Autodesk Fusion 360 part; units mm, degrees
(part 2 of 3)
sketch "Sketch3" plane through (0, -5, 0) normal (0, -1, 0) x (1, 0, 0)
  line L0 (28.5447, 14.3738) -> (28.5927, 14.6139)
  line L1 (28.5927, 14.6139) -> (28.6512, 39.9559)
  line L2 (28.6512, 39.9559) -> (28.9596, 41.1095)
  spline S0 degree 3 poles (28.9596, 41.1095) (29.1624, 41.8737) (29.4207, 42.6577) (29.7867, 43.4188) (30.0662, 43.9999) (30.3895, 44.5347) (30.7268, 45.0362) knots 0.002463 0.002463 0.002463 0.002463 0.566846 0.566846 0.566846 0.997755 0.997755 0.997755 0.997755
  spline S1 degree 3 poles (30.7268, 45.0362) (31.8623, 46.7358) (33.3627, 48.0126) (35.086, 48.9323) (35.8654, 49.3483) (36.6957, 49.6868) (37.5808, 49.9247) knots 0.001217 0.001217 0.001217 0.001217 0.688337 0.688337 0.688337 0.9991 0.9991 0.9991 0.9991
  spline S2 degree 3 poles (37.5809, 49.9247) (38.1393, 50.0755) (38.9538, 50.2376) (39.748, 50.2925) (40.2008, 50.3238) (40.6623, 50.3378) (41.2195, 50.3427) knots 0 0 0 0 0.456967 0.456967 0.456967 0.717487 0.717487 0.717487 0.717487
  line L3 (43.2375, 50.3785) -> (64.2895, 50.3304)
  spline S3 degree 3 poles (64.2895, 50.3304) (69.3375, 50.3217) (71.8718, 50.3178) (73.2853, 50.2995) (73.992, 50.2904) (74.4136, 50.2812) (74.8445, 50.2498) (75.1344, 50.2286) (75.4759, 50.185) (75.7431, 50.1318) (75.8658, 50.1074) (75.9593, 50.0853) (76.0131, 50.0726) knots 0 0 0 0 0.5 0.5 0.5 0.75 0.75 0.75 0.918213 0.918213 0.918213 0.99543 0.99543 0.99543 0.99543
  spline S4 degree 3 poles (76.0131, 50.0726) (78.7497, 49.4373) (81.2312, 47.9496) (82.9657, 45.7927) (83.8624, 44.6776) (84.5567, 43.3962) (85.0168, 42.022) (85.0171, 42.0211) (85.0175, 42.0201) (85.0178, 42.0192) knots 0.000788 0.000788 0.000788 0.000788 0.659473 0.659473 0.659473 1 1 1 1.000365 1.000365 1.000365 1.000365
  spline S5 degree 3 poles (85.0178, 42.0192) (85.0181, 42.0182) (85.0184, 42.0173) (85.0187, 42.0163) (85.0516, 41.9176) (85.1158, 41.7567) (85.2177, 41.4143) (85.3321, 41.0296) (85.439, 40.5049) (85.4918, 40.0367) (85.5914, 39.1525) (85.6029, 38.2865) (85.6162, 36.5721) (85.6311, 34.6649) (85.6279, 31.7431) (85.6279, 27.0233) knots -0.000791 -0.000791 -0.000791 -0.000791 0 0 0 0.151411 0.151411 0.151411 0.321524 0.321524 0.321524 0.642699 0.642699 0.642699 1 1 1 1
  spline S6 degree 3 poles (85.6279, 27.0233) (85.6279, 23.1991) (85.6318, 20.2771) (85.6408, 18.2245) (85.6454, 17.1759) (85.6514, 16.3534) (85.6586, 15.7622) (85.664, 15.321) (85.6707, 15.0001) (85.6757, 14.8547) (85.6761, 14.8429) (85.6765, 14.8324) (85.6768, 14.8233) knots 0 0 0 0 0.473518 0.473518 0.473518 0.715422 0.715422 0.715422 0.895914 0.895914 0.895914 0.91057 0.91057 0.91057 0.91057
  spline S7 degree 3 poles (85.6768, 14.8233) (85.78, 13.825) (86.1372, 12.4963) (86.5583, 11.5465) (86.6077, 11.435) (86.6576, 11.3286) (86.707, 11.2286) knots 0.016663 0.016663 0.016663 0.016663 0.893157 0.893157 0.893157 0.99609 0.99609 0.99609 0.99609
  spline S8 degree 3 poles (86.707, 11.2286) (87.0043, 10.6397) (87.1373, 10.444) (87.4643, 10.0658) (87.4655, 10.0645) (87.4666, 10.0631) (87.4678, 10.0618) knots 0.006764 0.006764 0.006764 0.006764 1 1 1 1.002067 1.002067 1.002067 1.002067
  spline S9 degree 3 poles (87.4678, 10.0618) (87.4689, 10.0605) (87.4701, 10.0591) (87.4712, 10.0578) (88.1686, 9.2476) (88.815, 8.3206) (89.28, 7.2967) (89.5333, 6.7388) (89.7284, 6.1697) (89.8772, 5.6188) (89.8788, 5.6129) (89.8804, 5.607) (89.882, 5.6011) knots -0.001455 -0.001455 -0.001455 -0.001455 0 0 0 0.647342 0.647342 0.647342 1 1 1 1.005845 1.005845 1.005845 1.005845
  spline S10 degree 3 poles (89.882, 5.6011) (89.8836, 5.5951) (89.8851, 5.5892) (89.8867, 5.5833) (89.9571, 5.3137) (90.0431, 4.9596) (90.1002, 4.5568) (90.1621, 4.1205) (90.1782, 3.7263) (90.185, 3.3701) (90.1876, 3.2384) (90.1889, 3.1062) (90.1899, 2.9643) (90.19, 2.959) (90.19, 2.9537) (90.19, 2.9484) knots -0.011583 -0.011583 -0.011583 -0.011583 0 0 0 0.402629 0.402629 0.402629 0.838702 0.838702 0.838702 1 1 1 1.006483 1.006483 1.006483 1.006483
  spline S11 degree 3 poles (90.19, 2.9484) (90.19, 2.9431) (90.19, 2.9377) (90.19, 2.9324) (90.19, 2.4687) (90.1909, 2.0734) (90.1389, 1.562) (90.0975, 1.1547) (90.0104, 0.7153) (89.9283, 0.3949) knots -0.006925 -0.006925 -0.006925 -0.006925 0 0 0 0.554445 0.554445 0.554445 0.995951 0.995951 0.995951 0.995951
  spline S12 degree 3 poles (89.9283, 0.3949) (89.2588, -2.2434) (87.6414, -4.4379) (85.5824, -5.8498) (83.3601, -7.3736) (80.5963, -8.0488) (77.8293, -7.5933) (76.6106, -7.3927) (75.3981, -6.9683) (74.2734, -6.3206) (74.2714, -6.3195) (74.2694, -6.3184) (74.2674, -6.3172) knots 0.000423 0.000423 0.000423 0.000423 0.3917 0.3917 0.3917 0.814004 0.814004 0.814004 1 1 1 1.000565 1.000565 1.000565 1.000565
  spline S13 degree 3 poles (74.2674, -6.3172) (74.2655, -6.316) (74.2635, -6.3149) (74.2615, -6.3137) (73.6843, -5.979) (72.7241, -5.6295) (71.6961, -5.4737) (71.6954, -5.4736) (71.6947, -5.4735) (71.694, -5.4734) knots -0.00171 -0.00171 -0.00171 -0.00171 0 0 0 1 1 1 1.000449 1.000449 1.000449 1.000449
  spline S14 degree 3 poles (71.694, -5.4734) (71.6933, -5.4733) (71.6927, -5.4732) (71.692, -5.4731) (71.4636, -5.4383) (71.3375, -5.4212) (70.8719, -5.3978) (69.9429, -5.351) (67.867, -5.3283) (63.1123, -5.3297) (61.2764, -5.3303) (59.0354, -5.3336) (56.2884, -5.3383) (56.2882, -5.3383) (56.2879, -5.3383) (56.2877, -5.3383) knots -0.000531 -0.000531 -0.000531 -0.000531 0 0 0 0.265563 0.265563 0.265563 0.795413 0.795413 0.795413 1 1 1 1.000016 1.000016 1.000016 1.000016
  spline S15 degree 3 poles (56.2877, -5.3383) (56.2875, -5.3383) (56.2873, -5.3383) (56.2871, -5.3383) (49.133, -5.3487) (45.769, -5.3576) (44.1594, -5.38) (43.3075, -5.3919) (42.958, -5.4118) (42.9119, -5.4159) (42.911, -5.416) (42.9103, -5.416) (42.9096, -5.4161) knots -0.000018 -0.000018 -0.000018 -0.000018 0 0 0 0.595196 0.595196 0.595196 0.910216 0.910216 0.910216 0.916088 0.916088 0.916088 0.916088
  spline S16 degree 3 poles (42.9096, -5.4161) (41.5575, -5.6043) (40.5785, -5.9576) (39.93, -6.3379) (39.9283, -6.3389) (39.9266, -6.3399) (39.9249, -6.3409) knots 0.005759 0.005759 0.005759 0.005759 1 1 1 1.001321 1.001321 1.001321 1.001321
  spline S17 degree 3 poles (39.9249, -6.3409) (39.9232, -6.3419) (39.9215, -6.3428) (39.9198, -6.3438) (38.3615, -7.2521) (36.7048, -7.6682) (34.9959, -7.7237) (34.5397, -7.7385) (34.079, -7.7249) (33.6144, -7.6795) knots -0.001663 -0.001663 -0.001663 -0.001663 0 0 0 0.789303 0.789303 0.789303 1 1 1 1
  spline S18 degree 3 poles (33.6144, -7.6795) (31.0087, -7.4269) (28.7159, -6.2217) (27.0024, -4.4425) (25.9971, -3.3987) (25.1834, -2.1388) (24.6669, -0.7013) (24.6659, -0.6984) (24.6649, -0.6956) (24.6639, -0.6927) knots 0.000439 0.000439 0.000439 0.000439 0.630416 0.630416 0.630416 1 1 1 1.001322 1.001322 1.001322 1.001322
  spline S19 degree 3 poles (24.6639, -0.6927) (23.792, 1.7499) (23.8315, 4.463) (24.7752, 6.841) (25.2611, 8.0655) (25.9744, 9.1996) (26.8664, 10.1907) (26.8665, 10.1908) (26.8666, 10.1909) (26.8668, 10.1911) knots 0 0 0 0 0.660104 0.660104 0.660104 1 1 1 1.000071 1.000071 1.000071 1.000071
  spline S20 degree 3 poles (26.8668, 10.1911) (26.8669, 10.1912) (26.867, 10.1913) (26.8671, 10.1914) (27.2467, 10.6131) (27.8393, 11.6247) (28.2707, 13.2034) (28.3696, 13.5653) (28.4615, 13.9552) (28.5441, 14.3711) (28.5443, 14.372) (28.5445, 14.3729) (28.5447, 14.3738) knots -0.000091 -0.000091 -0.000091 -0.000091 0 0 0 0.813499 0.813499 0.813499 1 1 1 1.000326 1.000326 1.000326 1.000326
  line L4 (28.1853, 41.3106) -> (27.8515, 40.0619)
  line L5 (27.8515, 40.0619) -> (27.7929, 14.694)
  line L6 (27.7929, 14.694) -> (27.7601, 14.5302)
  spline S21 degree 3 poles (27.7601, 14.5302) (27.7599, 14.5292) (27.7597, 14.5281) (27.7595, 14.5271) (27.6479, 13.9658) (27.5196, 13.4579) (27.3817, 13.0097) (26.9944, 11.7509) (26.5124, 10.993) (26.2726, 10.7267) (26.2725, 10.7266) (26.2723, 10.7264) (26.2722, 10.7263) knots -1.000384 -1.000384 -1.000384 -1.000384 -1 -1 -1 -0.737392 -0.737392 -0.737392 0 0 0 0.000107 0.000107 0.000107 0.000107
  spline S22 degree 3 poles (26.2722, 10.7263) (26.272, 10.7261) (26.2719, 10.726) (26.2718, 10.7258) (25.2452, 9.5852) (24.4359, 8.2609) (23.9141, 6.8271) (23.0115, 4.3472) (23.0138, 1.5501) (23.9104, -0.9616) (23.911, -0.9633) (23.9116, -0.965) (23.9122, -0.9667) knots -1.000083 -1.000083 -1.000083 -1.000083 -1 -1 -1 -0.633646 -0.633646 -0.633646 0 0 0 0.000763 0.000763 0.000763 0.000763
  spline S23 degree 3 poles (23.9122, -0.9667) (23.9128, -0.9684) (23.9134, -0.9701) (23.9141, -0.9718) (24.5193, -2.6566) (25.4993, -4.1093) (26.7116, -5.2837) (28.5164, -7.0321) (30.8677, -8.2168) (33.5366, -8.4758) knots -1.000779 -1.000779 -1.000779 -1.000779 -1 -1 -1 -0.598384 -0.598384 -0.598384 -0.000479 -0.000479 -0.000479 -0.000479
  spline S24 degree 3 poles (33.5366, -8.4758) (34.1121, -8.532) (34.6806, -8.5429) (35.2421, -8.5141) (36.9979, -8.4238) (38.6981, -7.9819) (40.3227, -7.035) (40.3247, -7.0338) (40.3267, -7.0327) (40.3287, -7.0315) knots -1 -1 -1 -1 -0.757667 -0.757667 -0.757667 0 0 0 0.001959 0.001959 0.001959 0.001959
  spline S25 degree 3 poles (40.3287, -7.0315) (40.3307, -7.0303) (40.3327, -7.0292) (40.3346, -7.028) (40.8689, -6.7147) (41.7382, -6.3892) (42.9969, -6.2117) knots -1.001555 -1.001555 -1.001555 -1.001555 -1 -1 -1 -0.011769 -0.011769 -0.011769 -0.011769
  spline S26 degree 3 poles (42.9969, -6.2117) (43.0795, -6.2058) (43.4713, -6.1887) (44.3196, -6.178) (45.9764, -6.157) (49.3494, -6.1484) (56.2883, -6.1383) (56.2885, -6.1383) (56.2888, -6.1383) (56.289, -6.1383) knots -0.872881 -0.872881 -0.872881 -0.872881 -0.57731 -0.57731 -0.57731 0 0 0 0.000021 0.000021 0.000021 0.000021
  spline S27 degree 3 poles (56.289, -6.1383) (56.2893, -6.1383) (56.2895, -6.1383) (56.2898, -6.1383) (59.3936, -6.1329) (61.8513, -6.1294) (63.8076, -6.1296) (68.0415, -6.1301) (69.9643, -6.1538) (70.8167, -6.196) (71.2742, -6.2187) (71.3614, -6.232) (71.5714, -6.264) (71.5722, -6.2641) (71.573, -6.2642) (71.5738, -6.2644) knots -1.000018 -1.000018 -1.000018 -1.000018 -1 -1 -1 -0.768828 -0.768828 -0.768828 -0.268512 -0.268512 -0.268512 0 0 0 0.000626 0.000626 0.000626 0.000626
  spline S28 degree 3 poles (71.5738, -6.2644) (71.5746, -6.2645) (71.5754, -6.2646) (71.5763, -6.2647) (72.5139, -6.4068) (73.3872, -6.7315) (73.8601, -7.0058) (73.8624, -7.0071) (73.8648, -7.0085) (73.8671, -7.0098) knots -1.000529 -1.000529 -1.000529 -1.000529 -1 -1 -1 0 0 0 0.002014 0.002014 0.002014 0.002014
  spline S29 degree 3 poles (73.8671, -7.0098) (73.8695, -7.0112) (73.8718, -7.0125) (73.8742, -7.0139) (75.2779, -7.8223) (76.8124, -8.3068) (78.3374, -8.4691) (81.2395, -8.778) (84.0823, -7.9571) (86.3566, -6.2808) (88.4137, -4.7645) (90.0207, -2.4927) (90.7035, 0.1972) knots -1.000666 -1.000666 -1.000666 -1.000666 -1 -1 -1 -0.783863 -0.783863 -0.783863 -0.372519 -0.372519 -0.372519 -0.000464 -0.000464 -0.000464 -0.000464
  spline S30 degree 3 poles (90.7035, 0.1972) (90.7945, 0.5524) (90.894, 1.0612) (90.9385, 1.5182) (90.9918, 2.0648) (90.99, 2.4724) (90.99, 2.9324) (90.99, 2.9387) (90.99, 2.945) (90.99, 2.9512) knots -0.995571 -0.995571 -0.995571 -0.995571 -0.542171 -0.542171 -0.542171 0 0 0 0.008156 0.008156 0.008156 0.008156
  spline S31 degree 3 poles (90.99, 2.9512) (90.99, 2.9575) (90.9899, 2.9637) (90.9899, 2.97) (90.9887, 3.1396) (90.9871, 3.2972) (90.9833, 3.46) (90.9752, 3.8126) (90.9554, 4.2319) (90.8895, 4.6883) (90.8262, 5.1272) (90.733, 5.5087) (90.6607, 5.7856) (90.6588, 5.7926) (90.657, 5.7996) (90.6552, 5.8065) knots -1.007635 -1.007635 -1.007635 -1.007635 -1 -1 -1 -0.809537 -0.809537 -0.809537 -0.396848 -0.396848 -0.396848 0 0 0 0.013642 0.013642 0.013642 0.013642
  spline S32 degree 3 poles (90.6552, 5.8065) (90.6533, 5.8135) (90.6514, 5.8205) (90.6495, 5.8275) (90.4769, 6.4667) (90.2416, 7.1395) (89.9313, 7.7935) (89.436, 8.8374) (88.7711, 9.7739) (88.0776, 10.5797) (88.0762, 10.5813) (88.0749, 10.5828) (88.0735, 10.5844) knots -1.006884 -1.006884 -1.006884 -1.006884 -1 -1 -1 -0.61483 -0.61483 -0.61483 0 0 0 0.001713 0.001713 0.001713 0.001713
  spline S33 degree 3 poles (88.0735, 10.5844) (88.0721, 10.586) (88.0708, 10.5876) (88.0694, 10.5891) (88.0403, 10.6228) (88.0135, 10.6546) (87.9887, 10.6847) (87.7701, 10.9505) (87.6698, 11.0971) (87.4227, 11.5861) knots -1.002435 -1.002435 -1.002435 -1.002435 -1 -1 -1 -0.898949 -0.898949 -0.898949 -0.008653 -0.008653 -0.008653 -0.008653
  spline S34 degree 3 poles (87.4227, 11.5861) (87.3635, 11.706) (87.3027, 11.838) (87.2426, 11.9789) (86.8785, 12.8313) (86.5675, 14.0165) (86.4753, 14.8796) knots -0.994911 -0.994911 -0.994911 -0.994911 -0.857358 -0.857358 -0.857358 -0.025015 -0.025015 -0.025015 -0.025015
  spline S35 degree 3 poles (86.4753, 14.8796) (86.4752, 14.8824) (86.4751, 14.8853) (86.475, 14.8883) (86.4703, 15.028) (86.4636, 15.3508) (86.4583, 15.7942) (86.4511, 16.388) (86.4452, 17.2152) (86.4406, 18.269) (86.4318, 20.3172) (86.4279, 23.225) (86.4279, 27.0233) knots -0.896967 -0.896967 -0.896967 -0.896967 -0.893105 -0.893105 -0.893105 -0.712378 -0.712378 -0.712378 -0.470371 -0.470371 -0.470371 0 0 0 0
  spline S36 degree 3 poles (86.4279, 27.0233) (86.4279, 32.0037) (86.4315, 34.9791) (86.4136, 36.8869) (86.3986, 38.4761) (86.3894, 39.3) (86.2734, 40.2394) (86.2125, 40.7327) (86.0879, 41.3033) (85.9679, 41.6972) (85.8632, 42.0409) (85.8042, 42.1896) (85.7777, 42.2693) (85.7773, 42.2704) (85.7769, 42.2715) (85.7766, 42.2727) knots -1 -1 -1 -1 -0.622947 -0.622947 -0.622947 -0.308857 -0.308857 -0.308857 -0.143922 -0.143922 -0.143922 0 0 0 0.000931 0.000931 0.000931 0.000931
  spline S37 degree 3 poles (85.7766, 42.2727) (85.7762, 42.2738) (85.7758, 42.2749) (85.7754, 42.276) (85.2484, 43.8501) (84.4288, 45.3154) (83.3624, 46.568) (81.5254, 48.7257) (78.9721, 50.2067) (76.1953, 50.8516) knots -1.00043 -1.00043 -1.00043 -1.00043 -1 -1 -1 -0.63304 -0.63304 -0.63304 -0.000881 -0.000881 -0.000881 -0.000881
  spline S38 degree 3 poles (76.1953, 50.8516) (76.1292, 50.8672) (75.9985, 50.898) (75.8301, 50.9298) (75.5363, 50.9854) (75.1922, 51.0265) (74.9027, 51.0476) (74.4377, 51.0816) (74.008, 51.0902) (73.2956, 51.0994) (71.8708, 51.1179) (69.3389, 51.1217) (64.2909, 51.1304) knots -0.994872 -0.994872 -0.994872 -0.994872 -0.905652 -0.905652 -0.905652 -0.75 -0.75 -0.75 -0.5 -0.5 -0.5 0 0 0 0
  line L7 (64.2909, 51.1304) -> (41.3067, 51.183)
  spline S39 degree 3 poles (40.09, 51.1135) (39.9226, 51.1058) (39.7579, 51.0959) (39.592, 51.0832) (38.7865, 51.022) (37.9297, 50.8475) (37.3724, 50.6971) knots -0.529015 -0.529015 -0.529015 -0.529015 -0.438651 -0.438651 -0.438651 0 0 0 0
  spline S40 degree 3 poles (37.3724, 50.6971) (36.3395, 50.4194) (35.3819, 50.0162) (34.4897, 49.5182) (32.7505, 48.5474) (31.2338, 47.2348) (30.0622, 45.4817) knots -0.999011 -0.999011 -0.999011 -0.999011 -0.660747 -0.660747 -0.660747 -0.001343 -0.001343 -0.001343 -0.001343
  spline S41 degree 3 poles (30.0622, 45.4817) (29.7101, 44.9579) (29.3636, 44.3856) (29.0632, 43.7602) (28.6708, 42.9432) (28.3952, 42.1024) (28.1853, 41.3106) knots -0.997484 -0.997484 -0.997484 -0.997484 -0.565614 -0.565614 -0.565614 -0.001492 -0.001492 -0.001492 -0.001492
  line L8 (42.0053, 0) -> (48.0053, 0)
  line L9 (48.0053, 0) -> (48.0053, -5.8307)
  line L10 (48.0053, -5.8307) -> (42.0053, -5.8307)
  line L11 (42.0053, -5.8307) -> (42.0053, 0)
  line L12 (72, 0) -> (66, 0)
  line L13 (66, 0) -> (66, -6)
  line L14 (66, -6) -> (72, -6)
  line L15 (72, -6) -> (72, 0)
  line L16 (80.6865, 13.92) -> (86.435, 13.92)
  line L17 (86.435, 13.92) -> (86.435, 19.92)
  line L18 (86.435, 19.92) -> (80.6865, 19.92)
  line L19 (80.6865, 19.92) -> (80.6865, 13.92)
  line L20 (80.6865, 38.9642) -> (86.1487, 38.9642)
  line L21 (86.1487, 38.9642) -> (86.1487, 32.9642)
  line L22 (86.1487, 32.9642) -> (80.6865, 32.9642)
  line L23 (80.6865, 32.9642) -> (80.6865, 38.9642)
  line L24 (74.3465, 45.2067) -> (68.3465, 45.2067)
  line L25 (68.3465, 45.2067) -> (68.3465, 50.5)
  line L26 (68.3465, 50.5) -> (74.3465, 50.5)
  line L27 (74.3465, 50.5) -> (74.3465, 45.2067)
  line L28 (54.0984, 45.8537) -> (60.0984, 45.8537)
  line L29 (60.0984, 45.8537) -> (60.0984, 50.5)
  line L30 (60.0984, 50.5) -> (54.0984, 50.5)
  line L31 (54.0984, 50.5) -> (54.0984, 45.8537)
  line L32 (45, 45.5) -> (39, 45.5)
  line L33 (39, 45.5) -> (39, 50.5)
  line L34 (39, 50.5) -> (45, 50.5)
  line L35 (45, 50.5) -> (45, 45.5)
  line L36 (34, 14.228) -> (28.2082, 14.228)
  line L37 (28.2082, 14.228) -> (28.2082, 20.228)
  line L38 (28.2082, 20.228) -> (34, 20.228)
  line L39 (34, 20.228) -> (34, 14.228)
  line L40 (33.5917, 38.2953) -> (28.2286, 38.2953)
  line L41 (28.2286, 38.2953) -> (28.2286, 32.2953)
  line L42 (28.2286, 32.2953) -> (33.5917, 32.2953)
  line L43 (33.5917, 32.2953) -> (33.5917, 38.2953)
  line L44 (41.2195, 50.3427) -> (43.2375, 50.3785)
  line L45 (41.3067, 51.183) -> (40.09, 51.1135)
  point P0 (54.0984, 45.8537)
  dimension "d7" = 6
  dimension "d8" = 6
  dimension "d9" = 6
  dimension "d10" = 6
  dimension "d11" = 6
  dimension "d12" = 6
  dimension "d13" = 6
  dimension "d14" = 6
  dimension "d15" = 6
  constraint horizontal L8
  constraint vertical L9
  constraint horizontal L10
  constraint vertical L11
  constraint horizontal L12
  constraint vertical L13
  constraint horizontal L14
  constraint vertical L15
  constraint horizontal L16
  constraint vertical L17
  constraint horizontal L18
  constraint vertical L19
  constraint coincident S35 L17.end
  constraint horizontal L20
  constraint vertical L21
  constraint horizontal L22
  constraint vertical L23
  constraint horizontal L24
  constraint vertical L25
  constraint horizontal L26
  constraint vertical L27
  constraint horizontal L28
  constraint vertical L29
  constraint horizontal L30
  constraint vertical L31
  constraint coincident P0 L28.start
  constraint horizontal L32
  constraint vertical L33
  constraint horizontal L34
  constraint vertical L35
  constraint horizontal L36
  constraint vertical L37
  constraint horizontal L38
  constraint vertical L39
  constraint horizontal L40
  constraint vertical L41
  constraint horizontal L42
  constraint vertical L43
  measures "d7" distance of L12.start L12.end
  measures "d8" distance of L8.start L8.end
  measures "d9" distance of L20.start L22.end
  measures "d10" distance of L16.end L17.end
  measures "d11" distance of L24.start L24.end
  measures "d12" distance of P0 L28.end
  measures "d13" distance of L32.start L32.end
  measures "d14" distance of L40.start L42.end
  measures "d15" distance of L36.start L38.end
extrude "Extrude3" add sketch "Sketch3" 1 faces at (81.3493, -5, 2.502) along normal blind 7 contours L0 L1 S20 L36 L37 L38 | L0 L1 S20 L36 L38 L39 | L4 L5 L6 S21 S22 S23 S24 S25 S26 S27 S28 S29 S30 S31 S32 S33 S34 S35 S36 S37 S38 L7 S39 S40 S41 L45 | L1 L40 L41 L42 | L1 L40 L42 L43 | S15 S16 L8 L9 L11 | S15 S16 L9 L10 L11 | S2 L3 L33 L34 L35 L44 | S2 L3 L32 L33 L35 L44 | S13 S14 L12 L13 L15 | S13 S14 L13 L14 L15 | L3 L29 L30 L31 | L3 L28 L29 L31 | S3 L25 L26 L27 | S3 L24 L25 L27 | S6 S7 L16 L18 L19 | S6 S7 L16 L17 L18 | S5 L20 L21 L22 | S5 L20 L22 L23 on bodies 3 bodies 2 3
sketch "Sketch6" plane through (0, -12, 0) normal (0, -1, 0) x (1, 0, 0)
  line L0 (33.1474, 38.2953) -> (28.6474, 38.2953)
  line L1 (28.6474, 38.2953) -> (28.6512, 39.9559)
  line L2 (28.6512, 39.9559) -> (28.9596, 41.1095)
  spline S0 degree 3 poles (28.9596, 41.1095) (29.1624, 41.8737) (29.4207, 42.6577) (29.7867, 43.4188) (30.0662, 43.9999) (30.3895, 44.5347) (30.7268, 45.0362) knots 0.002463 0.002463 0.002463 0.002463 0.566846 0.566846 0.566846 0.997755 0.997755 0.997755 0.997755
  spline S1 degree 3 poles (30.7268, 45.0362) (31.8623, 46.7358) (33.3627, 48.0126) (35.086, 48.9323) (35.8654, 49.3483) (36.6957, 49.6868) (37.5808, 49.9247) knots 0.001217 0.001217 0.001217 0.001217 0.688337 0.688337 0.688337 0.9991 0.9991 0.9991 0.9991
  spline S2 degree 3 poles (37.5809, 49.9247) (37.9634, 50.028) (38.466, 50.1366) (39, 50.2124) knots 0 0 0 0 0.313008 0.313008 0.313008 0.313008
  line L3 (39, 50.2124) -> (39, 45.6439)
  spline S3 degree 3 poles (39, 45.6439) (38.9203, 45.6244) (38.839, 45.6033) (38.7536, 45.5802) knots -0.090057 -0.090057 -0.090057 -0.090057 0 0 0 0
  spline S4 degree 3 poles (38.7536, 45.5802) (37.0603, 45.1263) (35.4193, 43.9625) (34.465, 42.531) knots -1 -1 -1 -1 0 0 0 0
  spline S5 degree 3 poles (34.465, 42.531) (33.8656, 41.6407) (33.5921, 41.0239) (33.307, 39.9474) knots -1 -1 -1 -1 0 0 0 0
  line L4 (33.307, 39.9474) -> (33.1499, 39.3597)
  line L5 (33.1499, 39.3597) -> (33.1474, 38.2953)
  line L6 (33.1335, 32.2953) -> (33.1057, 20.228)
  line L7 (33.1057, 20.228) -> (28.6057, 20.228)
  line L8 (28.6057, 20.228) -> (28.6335, 32.2953)
  line L9 (28.6335, 32.2953) -> (33.1335, 32.2953)
  line L10 (45, 45.8223) -> (45, 50.3745)
  line L11 (45, 50.3745) -> (54.0984, 50.3537)
  line L12 (54.0984, 50.3537) -> (54.0984, 45.8537)
  line L13 (54.0984, 45.8537) -> (60.0984, 45.8537)
  line L14 (60.0984, 45.8537) -> (60.0984, 50.34)
  line L15 (60.0984, 50.34) -> (64.2895, 50.3304)
  spline S6 degree 3 poles (64.2895, 50.3304) (65.8756, 50.3277) (67.2135, 50.3254) (68.3465, 50.323) knots 0 0 0 0 0.157099 0.157099 0.157099 0.157099
  line L16 (68.3465, 50.323) -> (68.3465, 45.8229)
  spline S7 degree 3 poles (68.3465, 45.8229) (67.2123, 45.8254) (65.8709, 45.8277) (64.2818, 45.8304) knots -0.157407 -0.157407 -0.157407 -0.157407 0 0 0 0
  line L17 (64.2818, 45.8304) -> (54.0984, 45.8537)
  line L18 (54.0984, 45.8537) -> (55.6987, 44.2477)
  line L19 (55.6987, 44.2477) -> (57.2989, 42.6474)
  line L20 (57.2989, 42.6474) -> (63.3391, 42.6474)
  line L21 (63.3391, 42.6474) -> (60.2608, 39.5517)
  spline S8 degree 3 poles (60.2608, 39.5517) (58.5733, 37.8467) (57.1651, 36.4385) (57.136, 36.4269) knots -1 -1 -1 -1 0 0 0 0
  spline S9 degree 3 poles (57.136, 36.4269) (57.1069, 36.4152) (55.1808, 38.3064) (52.8531, 40.6224) knots -1 -1 -1 -1 0 0 0 0
  spline S10 degree 3 poles (52.8531, 40.6224) (50.5313, 42.9442) (48.5063, 44.9285) (48.3492, 45.0274) knots -1 -1 -1 -1 0 0 0 0
  spline S11 degree 3 poles (48.3492, 45.0274) (47.9884, 45.2718) (47.4298, 45.5278) (46.9352, 45.685) knots -1 -1 -1 -1 0 0 0 0
  spline S12 degree 3 poles (46.9352, 45.685) (46.6336, 45.7809) (46.4863, 45.8051) (45, 45.8223) knots -1 -1 -1 -1 -0.214752 -0.214752 -0.214752 -0.214752
  line L22 (74.3465, 45.772) -> (74.3465, 50.277)
  spline S13 degree 3 poles (74.3465, 50.277) (74.5216, 50.2703) (74.6824, 50.2616) (74.8445, 50.2498) (75.1344, 50.2286) (75.4759, 50.185) (75.7431, 50.1318) (75.8658, 50.1074) (75.9593, 50.0853) (76.0131, 50.0726) knots 0.655951 0.655951 0.655951 0.655951 0.75 0.75 0.75 0.918213 0.918213 0.918213 0.99543 0.99543 0.99543 0.99543
  spline S14 degree 3 poles (76.0131, 50.0726) (78.7497, 49.4373) (81.2312, 47.9496) (82.9657, 45.7927) (83.8624, 44.6776) (84.5567, 43.3962) (85.0168, 42.022) (85.0171, 42.0211) (85.0175, 42.0201) (85.0178, 42.0192) knots 0.000788 0.000788 0.000788 0.000788 0.659473 0.659473 0.659473 1 1 1 1.000365 1.000365 1.000365 1.000365
  spline S15 degree 3 poles (85.0178, 42.0192) (85.0181, 42.0182) (85.0184, 42.0173) (85.0187, 42.0163) (85.0516, 41.9176) (85.1158, 41.7567) (85.2177, 41.4143) (85.3321, 41.0296) (85.439, 40.5049) (85.4918, 40.0367) (85.5305, 39.6934) (85.5559, 39.3528) (85.5733, 38.9642) knots -0.000791 -0.000791 -0.000791 -0.000791 0 0 0 0.151411 0.151411 0.151411 0.321524 0.321524 0.321524 0.446232 0.446232 0.446232 0.446232
  line L23 (85.5733, 38.9642) -> (81.0642, 38.9642)
  spline S16 degree 3 poles (81.0642, 38.9642) (81.0123, 39.9434) (80.9185, 40.0867) (80.7497, 40.5933) knots -0.420598 -0.420598 -0.420598 -0.420598 0 0 0 0
  spline S17 degree 3 poles (80.7497, 40.5933) (79.8768, 43.2002) (77.8052, 45.039) (74.9888, 45.6908) knots -1 -1 -1 -1 0 0 0 0
  spline S18 degree 3 poles (74.9888, 45.6908) (74.8321, 45.7278) (74.7143, 45.7535) (74.3465, 45.772) knots -1 -1 -1 -1 -0.697416 -0.697416 -0.697416 -0.697416
  line L24 (81.1275, 32.9642) -> (85.6275, 32.9642)
  spline S19 degree 3 poles (85.6275, 32.9642) (85.6287, 31.3852) (85.6279, 29.4399) (85.6279, 27.0233) knots 0.817055 0.817055 0.817055 0.817055 1 1 1 1
  spline S20 degree 3 poles (85.6279, 27.0233) (85.6279, 24.1513) (85.6301, 21.7882) (85.635, 19.92) knots 0 0 0 0 0.355613 0.355613 0.355613 0.355613
  line L25 (85.635, 19.92) -> (81.135, 19.92)
  spline S21 degree 3 poles (81.135, 19.92) (81.1301, 21.793) (81.1279, 24.1549) (81.1279, 27.0233) knots -0.354876 -0.354876 -0.354876 -0.354876 0 0 0 0
  spline S22 degree 3 poles (81.1279, 27.0233) (81.1279, 29.4417) (81.1287, 31.3891) (81.1275, 32.9642) knots -1 -1 -1 -1 -0.816995 -0.816995 -0.816995 -0.816995
  line L26 (81.2537, 13.92) -> (85.8196, 13.92)
  spline S23 degree 3 poles (85.8196, 13.92) (85.9856, 13.1087) (86.2554, 12.2296) (86.5583, 11.5465) (86.6077, 11.435) (86.6576, 11.3286) (86.707, 11.2286) knots 0.262747 0.262747 0.262747 0.262747 0.893157 0.893157 0.893157 0.99609 0.99609 0.99609 0.99609
  spline S24 degree 3 poles (86.707, 11.2286) (87.0043, 10.6397) (87.1373, 10.444) (87.4643, 10.0658) (87.4655, 10.0645) (87.4666, 10.0631) (87.4678, 10.0618) knots 0.006764 0.006764 0.006764 0.006764 1 1 1 1.002067 1.002067 1.002067 1.002067
  spline S25 degree 3 poles (87.4678, 10.0618) (87.4689, 10.0605) (87.4701, 10.0591) (87.4712, 10.0578) (88.1686, 9.2476) (88.815, 8.3206) (89.28, 7.2967) (89.5333, 6.7388) (89.7284, 6.1697) (89.8772, 5.6188) (89.8788, 5.6129) (89.8804, 5.607) (89.882, 5.6011) knots -0.001455 -0.001455 -0.001455 -0.001455 0 0 0 0.647342 0.647342 0.647342 1 1 1 1.005845 1.005845 1.005845 1.005845
  spline S26 degree 3 poles (89.882, 5.6011) (89.8836, 5.5951) (89.8851, 5.5892) (89.8867, 5.5833) (89.9571, 5.3137) (90.0431, 4.9596) (90.1002, 4.5568) (90.1621, 4.1205) (90.1782, 3.7263) (90.185, 3.3701) (90.1876, 3.2384) (90.1889, 3.1062) (90.1899, 2.9643) (90.19, 2.959) (90.19, 2.9537) (90.19, 2.9484) knots -0.011583 -0.011583 -0.011583 -0.011583 0 0 0 0.402629 0.402629 0.402629 0.838702 0.838702 0.838702 1 1 1 1.006483 1.006483 1.006483 1.006483
  spline S27 degree 3 poles (90.19, 2.9484) (90.19, 2.9431) (90.19, 2.9377) (90.19, 2.9324) (90.19, 2.4687) (90.1909, 2.0734) (90.1389, 1.562) (90.0975, 1.1547) (90.0104, 0.7153) (89.9283, 0.3949) knots -0.006925 -0.006925 -0.006925 -0.006925 0 0 0 0.554445 0.554445 0.554445 0.995951 0.995951 0.995951 0.995951
  spline S28 degree 3 poles (89.9283, 0.3949) (89.2588, -2.2434) (87.6414, -4.4379) (85.5824, -5.8498) (83.3601, -7.3736) (80.5963, -8.0488) (77.8293, -7.5933) (76.6106, -7.3927) (75.3981, -6.9683) (74.2734, -6.3206) (74.2714, -6.3195) (74.2694, -6.3184) (74.2674, -6.3172) knots 0.000423 0.000423 0.000423 0.000423 0.3917 0.3917 0.3917 0.814004 0.814004 0.814004 1 1 1 1.000565 1.000565 1.000565 1.000565
  spline S29 degree 3 poles (74.2674, -6.3172) (74.2655, -6.316) (74.2635, -6.3149) (74.2615, -6.3137) (73.7416, -6.0122) (72.911, -5.6988) (72, -5.5257) knots -0.00171 -0.00171 -0.00171 -0.00171 0 0 0 0.90071 0.90071 0.90071 0.90071
  line L27 (72, -5.5257) -> (72, -0.9744)
  spline S30 degree 3 poles (72, -0.9744) (72.1302, -0.9896) (72.2505, -1.0063) (72.3702, -1.0245) knots -0.092261 -0.092261 -0.092261 -0.092261 0 0 0 0
  spline S31 degree 3 poles (72.3702, -1.0245) (73.9065, -1.2573) (75.3554, -1.7461) (76.5192, -2.4211) knots -1 -1 -1 -1 0 0 0 0
  spline S32 degree 3 poles (76.5192, -2.4211) (80.0456, -4.4519) (84.5553, -2.4967) (85.5678, 1.5068) knots -1 -1 -1 -1 0 0 0 0
  spline S33 degree 3 poles (85.5678, 1.5068) (85.6726, 1.9141) (85.69, 2.1643) (85.69, 2.9324) knots -1 -1 -1 -1 0 0 0 0
  spline S34 degree 3 poles (85.69, 2.9324) (85.6842, 3.7529) (85.6668, 3.9333) (85.5329, 4.4454) knots -1 -1 -1 -1 0 0 0 0
  spline S35 degree 3 poles (85.5329, 4.4454) (85.2594, 5.4579) (84.8521, 6.2027) (84.0607, 7.1221) knots -1 -1 -1 -1 0 0 0 0
  spline S36 degree 3 poles (84.0607, 7.1221) (83.5021, 7.768) (83.1006, 8.3849) (82.6816, 9.217) knots -1 -1 -1 -1 0 0 0 0
  spline S37 degree 3 poles (82.6816, 9.217) (81.9952, 10.6003) (81.4739, 12.3138) (81.2537, 13.92) knots -1 -1 -1 -1 -0.099571 -0.099571 -0.099571 -0.099571
  line L28 (66, -0.832) -> (66, -5.3326)
  spline S38 degree 3 poles (66, -5.3326) (65.1681, -5.3304) (64.2118, -5.3294) (63.1123, -5.3297) (61.2764, -5.3303) (59.0354, -5.3336) (56.2884, -5.3383) (56.2882, -5.3383) (56.2879, -5.3383) (56.2877, -5.3383) knots 0.672886 0.672886 0.672886 0.672886 0.795413 0.795413 0.795413 1 1 1 1.000016 1.000016 1.000016 1.000016
  spline S39 degree 3 poles (56.2877, -5.3383) (56.2875, -5.3383) (56.2873, -5.3383) (56.2871, -5.3383) (52.6239, -5.3436) (49.9544, -5.3486) (48.0053, -5.3551) knots -0.000018 -0.000018 -0.000018 -0.000018 0 0 0 0.304767 0.304767 0.304767 0.304767
  line L29 (48.0053, -5.3551) -> (48.0053, -0.8549)
  spline S40 degree 3 poles (48.0053, -0.8549) (49.9594, -0.8484) (52.6228, -0.8436) (56.2806, -0.8383) knots -0.304255 -0.304255 -0.304255 -0.304255 0 0 0 0
  spline S41 degree 3 poles (56.2806, -0.8383) (60.6697, -0.8307) (63.7698, -0.8268) (66, -0.832) knots -1 -1 -1 -1 -0.673196 -0.673196 -0.673196 -0.673196
  spline S42 degree 3 poles (57.5317, 2.3505) (52.0618, 2.3389) (47.3192, 2.3563) (46.9992, 2.3796) knots -1 -1 -1 -1 0 0 0 0
  spline S43 degree 3 poles (46.9992, 2.3796) (46.2718, 2.4378) (45.0673, 2.6822) (44.3806, 2.9091) knots -1 -1 -1 -1 0 0 0 0
  spline S44 degree 3 poles (44.3806, 2.9091) (43.6474, 3.1477) (42.3265, 3.8227) (41.7039, 4.265) knots -1 -1 -1 -1 0 0 0 0
  spline S45 degree 3 poles (41.7039, 4.265) (41.0347, 4.748) (40.1967, 5.5277) (39.6614, 6.1736) knots -1 -1 -1 -1 0 0 0 0
  spline S46 degree 3 poles (39.6614, 6.1736) (38.5383, 7.5178) (37.6363, 9.217) (37.0253, 11.1373) knots -1 -1 -1 -1 0 0 0 0
  line L30 (37.0253, 11.1373) -> (36.8391, 11.7134)
  line L31 (36.8391, 11.7134) -> (46.6791, 21.5534)
  line L32 (46.6791, 21.5534) -> (49.7516, 18.4809)
  line L33 (49.7516, 18.4809) -> (50.0076, 18.574)
  spline S47 degree 3 poles (50.0076, 18.574) (50.7467, 18.8592) (52.8008, 19.7611) (52.8008, 19.8018) knots -1 -1 -1 -1 0 0 0 0
  spline S48 degree 3 poles (52.8008, 19.8018) (52.8008, 19.8251) (49.8505, 22.8045) (46.2485, 26.4181) knots -1 -1 -1 -1 0 0 0 0
  line L34 (46.2485, 26.4181) -> (39.6963, 32.9936)
  line L35 (39.6963, 32.9936) -> (39.6963, 28.5944)
  line L36 (39.6963, 28.5944) -> (42.0821, 26.2086)
  spline S49 degree 3 poles (42.0821, 26.2086) (43.3972, 24.8993) (44.4679, 23.7995) (44.4679, 23.7646) knots -1 -1 -1 -1 0 0 0 0
  spline S50 degree 3 poles (44.4679, 23.7646) (44.4679, 23.6948) (36.4318, 15.647) (36.362, 15.647) knots -1 -1 -1 -1 0 0 0 0
  spline S51 degree 3 poles (36.362, 15.647) (36.3387, 15.647) (36.3271, 20.9191) (36.3329, 27.355) knots -1 -1 -1 -1 0 0 0 0
  line L37 (36.3329, 27.355) -> (36.3503, 39.0687)
  line L38 (36.3503, 39.0687) -> (36.5133, 39.5342)
  spline S52 degree 3 poles (36.5133, 39.5342) (36.9497, 40.7679) (37.7062, 41.6465) (38.7943, 42.1877) knots -1 -1 -1 -1 0 0 0 0
  spline S53 degree 3 poles (38.7943, 42.1877) (39.7196, 42.6416) (39.8068, 42.6532) (43.1353, 42.6358) knots -1 -1 -1 -1 0 0 0 0
  line L39 (43.1353, 42.6358) -> (46.0681, 42.6183)
  line L40 (46.0681, 42.6183) -> (46.4464, 42.4496)
  spline S54 degree 3 poles (46.4464, 42.4496) (46.8013, 42.2866) (47.0923, 42.0131) (50.8572, 38.2599) knots -1 -1 -1 -1 0 0 0 0
  spline S55 degree 3 poles (50.8572, 38.2599) (53.0685, 36.0486) (54.884, 34.2156) (54.884, 34.1807) knots -1 -1 -1 -1 0 0 0 0
  spline S56 degree 3 poles (54.884, 34.1807) (54.884, 34.1516) (54.0693, 33.3078) (53.0685, 32.307) knots -1 -1 -1 -1 0 0 0 0
  line L41 (53.0685, 32.307) -> (51.2587, 30.4972)
  line L42 (51.2587, 30.4972) -> (51.7883, 29.252)
  spline S57 degree 3 poles (51.7883, 29.252) (52.0792, 28.5711) (52.3702, 27.8845) (52.44, 27.7274) knots -1 -1 -1 -1 0 0 0 0
  line L43 (52.44, 27.7274) -> (52.5622, 27.4364)
  line L44 (52.5622, 27.4364) -> (57.1243, 31.9986)
  line L45 (57.1243, 31.9986) -> (65.3292, 23.7937)
  line L46 (65.3292, 23.7937) -> (58.2765, 16.7352)
  line L47 (58.2765, 16.7352) -> (51.2238, 9.6825)
  line L48 (51.2238, 9.6825) -> (51.8581, 8.1987)
  spline S58 degree 3 poles (51.8581, 8.1987) (52.2072, 7.384) (52.504, 6.6857) (52.5215, 6.6566) knots -1 -1 -1 -1 0 0 0 0
  spline S59 degree 3 poles (52.5215, 6.6566) (52.5331, 6.6217) (53.5631, 7.6109) (54.8025, 8.8504) knots -1 -1 -1 -1 0 0 0 0
  spline S60 degree 3 poles (54.8025, 8.8504) (56.0478, 10.0957) (57.0952, 11.1082) (57.1301, 11.1082) knots -1 -1 -1 -1 0 0 0 0
  spline S61 degree 3 poles (57.1301, 11.1082) (57.1651, 11.1082) (58.4045, 9.892) (59.8767, 8.4023) knots -1 -1 -1 -1 0 0 0 0
  line L49 (59.8767, 8.4023) -> (62.5651, 5.6965)
  line L50 (62.5651, 5.6965) -> (63.7522, 5.6965)
  spline S62 degree 3 poles (63.7522, 5.6965) (64.3981, 5.6965) (65.3699, 5.7139) (65.9053, 5.7372) knots -1 -1 -1 -1 0 0 0 0
  line L51 (65.9053, 5.7372) -> (66.8829, 5.7721)
  line L52 (66.8829, 5.7721) -> (59.3065, 13.3485)
  line L53 (59.3065, 13.3485) -> (74.5524, 28.5944)
  line L54 (74.5524, 28.5944) -> (74.5524, 32.9936)
  line L55 (74.5524, 32.9936) -> (71.0551, 29.5138)
  spline S63 degree 3 poles (71.0551, 29.5138) (69.1348, 27.5994) (67.5462, 26.0282) (67.523, 26.0166) knots -1 -1 -1 -1 0 0 0 0
  spline S64 degree 3 poles (67.523, 26.0166) (67.4997, 26.0108) (65.6434, 27.8438) (63.3914, 30.0957) knots -1 -1 -1 -1 0 0 0 0
  line L56 (63.3914, 30.0957) -> (59.3065, 34.1807)
  line L57 (59.3065, 34.1807) -> (67.779, 42.6532)
  line L58 (67.779, 42.6532) -> (71.09, 42.6358)
  line L59 (71.09, 42.6358) -> (74.4069, 42.6183)
  line L60 (74.4069, 42.6183) -> (74.919, 42.4379)
  spline S65 degree 3 poles (74.919, 42.4379) (76.5599, 41.8502) (77.6888, 40.4769) (77.9216, 38.7836) knots -1 -1 -1 -1 0 0 0 0
  spline S66 degree 3 poles (77.9216, 38.7836) (77.9972, 38.2599) (78.0147, 15.5888) (77.9391, 15.5888) knots -1 -1 -1 -1 0 0 0 0
  spline S67 degree 3 poles (77.9391, 15.5888) (77.9158, 15.5888) (77.0837, 16.3977) (76.0944, 17.3928) knots -1 -1 -1 -1 0 0 0 0
  spline S68 degree 3 poles (76.0944, 17.3928) (75.1052, 18.382) (74.2731, 19.1967) (74.244, 19.1967) knots -1 -1 -1 -1 0 0 0 0
  spline S69 degree 3 poles (74.244, 19.1967) (74.2032, 19.1967) (71.5206, 18.0619) (71.3286, 17.963) knots -1 -1 -1 -1 0 0 0 0
  spline S70 degree 3 poles (71.3286, 17.963) (71.2355, 17.9106) (71.6079, 17.515) (74.3254, 14.7975) knots -1 -1 -1 -1 0 0 0 0
  line L61 (74.3254, 14.7975) -> (77.427, 11.6959)
  line L62 (77.427, 11.6959) -> (77.3513, 11.3875)
  spline S71 degree 3 poles (77.3513, 11.3875) (77.0778, 10.2993) (76.2283, 8.4547) (75.4951, 7.3549) knots -1 -1 -1 -1 0 0 0 0
  spline S72 degree 3 poles (75.4951, 7.3549) (73.6388, 4.5676) (71.2995, 3.0372) (68.0292, 2.4553) knots -1 -1 -1 -1 0 0 0 0
  spline S73 degree 3 poles (68.0292, 2.4553) (67.5346, 2.368) (66.5046, 2.3563) (57.5317, 2.3505) knots -1 -1 -1 -1 0 0 0 0
  line L63 (33.0918, 14.228) -> (33.0917, 14.1632)
  line L64 (33.0917, 14.1632) -> (32.9578, 13.494)
  spline S74 degree 3 poles (32.9578, 13.494) (32.4108, 10.7416) (31.474, 8.5827) (30.2112, 7.1803) knots -1 -1 -1 -1 0 0 0 0
  spline S75 degree 3 poles (30.2112, 7.1803) (28.5877, 5.3764) (28.1106, 3.0372) (28.902, 0.8201) knots -1 -1 -1 -1 0 0 0 0
  spline S76 degree 3 poles (28.902, 0.8201) (29.6817, -1.3504) (31.7591, -2.9797) (34.0518, -3.2009) knots -1 -1 -1 -1 0 0 0 0
  spline S77 degree 3 poles (34.0518, -3.2009) (35.3029, -3.3231) (36.6355, -3.0496) (37.6538, -2.456) knots -1 -1 -1 -1 0 0 0 0
  spline S78 degree 3 poles (37.6538, -2.456) (38.8595, -1.749) (40.3181, -1.264) (42.0053, -1.0009) knots -1 -1 -1 -1 -0.058189 -0.058189 -0.058189 -0.058189
  line L65 (42.0053, -1.0009) -> (42.0053, -5.577)
  spline S79 degree 3 poles (42.0053, -5.577) (41.1093, -5.7743) (40.4239, -6.0483) (39.93, -6.3379) (39.9283, -6.3389) (39.9266, -6.3399) (39.9249, -6.3409) knots 0.242864 0.242864 0.242864 0.242864 1 1 1 1.001321 1.001321 1.001321 1.001321
  spline S80 degree 3 poles (39.9249, -6.3409) (39.9232, -6.3419) (39.9215, -6.3428) (39.9198, -6.3438) (38.3615, -7.2521) (36.7048, -7.6682) (34.9959, -7.7237) (34.5397, -7.7385) (34.079, -7.7249) (33.6144, -7.6795) knots -0.001663 -0.001663 -0.001663 -0.001663 0 0 0 0.789303 0.789303 0.789303 1 1 1 1
  spline S81 degree 3 poles (33.6144, -7.6795) (31.0087, -7.4269) (28.7159, -6.2217) (27.0024, -4.4425) (25.9971, -3.3987) (25.1834, -2.1388) (24.6669, -0.7013) (24.6659, -0.6984) (24.6649, -0.6956) (24.6639, -0.6927) knots 0.000439 0.000439 0.000439 0.000439 0.630416 0.630416 0.630416 1 1 1 1.001322 1.001322 1.001322 1.001322
  spline S82 degree 3 poles (24.6639, -0.6927) (23.792, 1.7499) (23.8315, 4.463) (24.7752, 6.841) (25.2611, 8.0655) (25.9744, 9.1996) (26.8664, 10.1907) (26.8665, 10.1908) (26.8666, 10.1909) (26.8668, 10.1911) knots 0 0 0 0 0.660104 0.660104 0.660104 1 1 1 1.000071 1.000071 1.000071 1.000071
  spline S83 degree 3 poles (26.8668, 10.1911) (26.8669, 10.1912) (26.867, 10.1913) (26.8671, 10.1914) (27.2467, 10.6131) (27.8393, 11.6247) (28.2707, 13.2034) (28.3582, 13.5235) (28.4402, 13.8655) (28.5151, 14.228) knots -0.000091 -0.000091 -0.000091 -0.000091 0 0 0 0.813499 0.813499 0.813499 0.97845 0.97845 0.97845 0.97845
  line L66 (28.5151, 14.228) -> (33.0918, 14.228)
  spline S84 degree 3 poles (86.435, 19.92) (86.4301, 21.7873) (86.4279, 24.1506) (86.4279, 27.0233) knots -0.355745 -0.355745 -0.355745 -0.355745 0 0 0 0
  spline S85 degree 3 poles (86.4279, 27.0233) (86.4279, 32.0037) (86.4315, 34.9791) (86.4136, 36.8869) (86.3986, 38.4761) (86.3894, 39.3) (86.2734, 40.2394) (86.2125, 40.7327) (86.0879, 41.3033) (85.9679, 41.6972) (85.8632, 42.0409) (85.8042, 42.1896) (85.7777, 42.2693) (85.7773, 42.2704) (85.7769, 42.2715) (85.7766, 42.2727) knots -1 -1 -1 -1 -0.622947 -0.622947 -0.622947 -0.308857 -0.308857 -0.308857 -0.143922 -0.143922 -0.143922 0 0 0 0.000931 0.000931 0.000931 0.000931
  spline S86 degree 3 poles (85.7766, 42.2727) (85.7762, 42.2738) (85.7758, 42.2749) (85.7754, 42.276) (85.2484, 43.8501) (84.4288, 45.3154) (83.3624, 46.568) (81.5254, 48.7257) (78.9721, 50.2067) (76.1953, 50.8516) knots -1.00043 -1.00043 -1.00043 -1.00043 -1 -1 -1 -0.63304 -0.63304 -0.63304 -0.000881 -0.000881 -0.000881 -0.000881
  spline S87 degree 3 poles (76.1953, 50.8516) (76.1292, 50.8672) (75.9985, 50.898) (75.8301, 50.9298) (75.5363, 50.9854) (75.1922, 51.0265) (74.9027, 51.0476) (74.4377, 51.0816) (74.008, 51.0902) (73.2956, 51.0994) (71.8708, 51.1179) (69.3389, 51.1217) (64.2909, 51.1304) knots -0.994872 -0.994872 -0.994872 -0.994872 -0.905652 -0.905652 -0.905652 -0.75 -0.75 -0.75 -0.5 -0.5 -0.5 0 0 0 0
  line L67 (64.2909, 51.1304) -> (41.3067, 51.183)
  line L68 (41.3067, 51.183) -> (40.09, 51.1135)
  spline S88 degree 3 poles (40.09, 51.1135) (39.9226, 51.1058) (39.7579, 51.0959) (39.592, 51.0832) (38.7865, 51.022) (37.9297, 50.8475) (37.3724, 50.6971) knots -0.529015 -0.529015 -0.529015 -0.529015 -0.438651 -0.438651 -0.438651 0 0 0 0
  spline S89 degree 3 poles (37.3724, 50.6971) (36.3395, 50.4194) (35.3819, 50.0162) (34.4897, 49.5182) (32.7505, 48.5474) (31.2338, 47.2348) (30.0622, 45.4817) knots -0.999011 -0.999011 -0.999011 -0.999011 -0.660747 -0.660747 -0.660747 -0.001343 -0.001343 -0.001343 -0.001343
  spline S90 degree 3 poles (30.0622, 45.4817) (29.7101, 44.9579) (29.3636, 44.3856) (29.0632, 43.7602) (28.6708, 42.9432) (28.3952, 42.1024) (28.1853, 41.3106) knots -0.997484 -0.997484 -0.997484 -0.997484 -0.565614 -0.565614 -0.565614 -0.001492 -0.001492 -0.001492 -0.001492
  line L69 (28.1853, 41.3106) -> (27.8515, 40.0619)
  line L70 (27.8515, 40.0619) -> (27.7929, 14.694)
  line L71 (27.7929, 14.694) -> (27.7601, 14.5302)
  spline S91 degree 3 poles (27.7601, 14.5302) (27.7599, 14.5292) (27.7597, 14.5281) (27.7595, 14.5271) (27.6479, 13.9658) (27.5196, 13.4579) (27.3817, 13.0097) (26.9944, 11.7509) (26.5124, 10.993) (26.2726, 10.7267) (26.2725, 10.7266) (26.2723, 10.7264) (26.2722, 10.7263) knots -1.000384 -1.000384 -1.000384 -1.000384 -1 -1 -1 -0.737392 -0.737392 -0.737392 0 0 0 0.000107 0.000107 0.000107 0.000107
  spline S92 degree 3 poles (26.2722, 10.7263) (26.272, 10.7261) (26.2719, 10.726) (26.2718, 10.7258) (25.2452, 9.5852) (24.4359, 8.2609) (23.9141, 6.8271) (23.0115, 4.3472) (23.0138, 1.5501) (23.9104, -0.9616) (23.911, -0.9633) (23.9116, -0.965) (23.9122, -0.9667) knots -1.000083 -1.000083 -1.000083 -1.000083 -1 -1 -1 -0.633646 -0.633646 -0.633646 0 0 0 0.000763 0.000763 0.000763 0.000763
  spline S93 degree 3 poles (23.9122, -0.9667) (23.9128, -0.9684) (23.9134, -0.9701) (23.9141, -0.9718) (24.5193, -2.6566) (25.4993, -4.1093) (26.7116, -5.2837) (28.5164, -7.0321) (30.8677, -8.2168) (33.5366, -8.4758) knots -1.000779 -1.000779 -1.000779 -1.000779 -1 -1 -1 -0.598384 -0.598384 -0.598384 -0.000479 -0.000479 -0.000479 -0.000479
  spline S94 degree 3 poles (33.5366, -8.4758) (34.1121, -8.532) (34.6806, -8.5429) (35.2421, -8.5141) (36.9979, -8.4238) (38.6981, -7.9819) (40.3227, -7.035) (40.3247, -7.0338) (40.3267, -7.0327) (40.3287, -7.0315) knots -1 -1 -1 -1 -0.757667 -0.757667 -0.757667 0 0 0 0.001959 0.001959 0.001959 0.001959
  spline S95 degree 3 poles (40.3287, -7.0315) (40.3307, -7.0303) (40.3327, -7.0292) (40.3346, -7.028) (40.8689, -6.7147) (41.7382, -6.3892) (42.9969, -6.2117) knots -1.001555 -1.001555 -1.001555 -1.001555 -1 -1 -1 -0.011769 -0.011769 -0.011769 -0.011769
  spline S96 degree 3 poles (42.9969, -6.2117) (43.0795, -6.2058) (43.4713, -6.1887) (44.3196, -6.178) (45.9764, -6.157) (49.3494, -6.1484) (56.2883, -6.1383) (56.2885, -6.1383) (56.2888, -6.1383) (56.289, -6.1383) knots -0.872881 -0.872881 -0.872881 -0.872881 -0.57731 -0.57731 -0.57731 0 0 0 0.000021 0.000021 0.000021 0.000021
  spline S97 degree 3 poles (56.289, -6.1383) (56.2893, -6.1383) (56.2895, -6.1383) (56.2898, -6.1383) (59.3936, -6.1329) (61.8513, -6.1294) (63.8076, -6.1296) (68.0415, -6.1301) (69.9643, -6.1538) (70.8167, -6.196) (71.2742, -6.2187) (71.3614, -6.232) (71.5714, -6.264) (71.5722, -6.2641) (71.573, -6.2642) (71.5738, -6.2644) knots -1.000018 -1.000018 -1.000018 -1.000018 -1 -1 -1 -0.768828 -0.768828 -0.768828 -0.268512 -0.268512 -0.268512 0 0 0 0.000626 0.000626 0.000626 0.000626
  spline S98 degree 3 poles (71.5738, -6.2644) (71.5746, -6.2645) (71.5754, -6.2646) (71.5763, -6.2647) (72.5139, -6.4068) (73.3872, -6.7315) (73.8601, -7.0058) (73.8624, -7.0071) (73.8648, -7.0085) (73.8671, -7.0098) knots -1.000529 -1.000529 -1.000529 -1.000529 -1 -1 -1 0 0 0 0.002014 0.002014 0.002014 0.002014
  spline S99 degree 3 poles (73.8671, -7.0098) (73.8695, -7.0112) (73.8718, -7.0125) (73.8742, -7.0139) (75.2779, -7.8223) (76.8124, -8.3068) (78.3374, -8.4691) (81.2395, -8.778) (84.0823, -7.9571) (86.3566, -6.2808) (88.4137, -4.7645) (90.0207, -2.4927) (90.7035, 0.1972) knots -1.000666 -1.000666 -1.000666 -1.000666 -1 -1 -1 -0.783863 -0.783863 -0.783863 -0.372519 -0.372519 -0.372519 -0.000464 -0.000464 -0.000464 -0.000464
  spline S100 degree 3 poles (90.7035, 0.1972) (90.7945, 0.5524) (90.894, 1.0612) (90.9385, 1.5182) (90.9918, 2.0648) (90.99, 2.4724) (90.99, 2.9324) (90.99, 2.9387) (90.99, 2.945) (90.99, 2.9512) knots -0.995571 -0.995571 -0.995571 -0.995571 -0.542171 -0.542171 -0.542171 0 0 0 0.008156 0.008156 0.008156 0.008156
  spline S101 degree 3 poles (90.99, 2.9512) (90.99, 2.9575) (90.9899, 2.9637) (90.9899, 2.97) (90.9887, 3.1396) (90.9871, 3.2972) (90.9833, 3.46) (90.9752, 3.8126) (90.9554, 4.2319) (90.8895, 4.6883) (90.8262, 5.1272) (90.733, 5.5087) (90.6607, 5.7856) (90.6588, 5.7926) (90.657, 5.7996) (90.6552, 5.8065) knots -1.007635 -1.007635 -1.007635 -1.007635 -1 -1 -1 -0.809537 -0.809537 -0.809537 -0.396848 -0.396848 -0.396848 0 0 0 0.013642 0.013642 0.013642 0.013642
  spline S102 degree 3 poles (90.6552, 5.8065) (90.6533, 5.8135) (90.6514, 5.8205) (90.6495, 5.8275) (90.4769, 6.4667) (90.2416, 7.1395) (89.9313, 7.7935) (89.436, 8.8374) (88.7711, 9.7739) (88.0776, 10.5797) (88.0762, 10.5813) (88.0749, 10.5828) (88.0735, 10.5844) knots -1.006884 -1.006884 -1.006884 -1.006884 -1 -1 -1 -0.61483 -0.61483 -0.61483 0 0 0 0.001713 0.001713 0.001713 0.001713
  spline S103 degree 3 poles (88.0735, 10.5844) (88.0721, 10.586) (88.0708, 10.5876) (88.0694, 10.5891) (88.0403, 10.6228) (88.0135, 10.6546) (87.9887, 10.6847) (87.7701, 10.9505) (87.6698, 11.0971) (87.4227, 11.5861) knots -1.002435 -1.002435 -1.002435 -1.002435 -1 -1 -1 -0.898949 -0.898949 -0.898949 -0.008653 -0.008653 -0.008653 -0.008653
  spline S104 degree 3 poles (87.4227, 11.5861) (87.3635, 11.706) (87.3027, 11.838) (87.2426, 11.9789) (86.8785, 12.8313) (86.5675, 14.0165) (86.4753, 14.8796) knots -0.994911 -0.994911 -0.994911 -0.994911 -0.857358 -0.857358 -0.857358 -0.025015 -0.025015 -0.025015 -0.025015
  spline S105 degree 3 poles (86.4753, 14.8796) (86.4752, 14.8824) (86.4751, 14.8853) (86.475, 14.8883) (86.4703, 15.028) (86.4636, 15.3508) (86.4583, 15.7942) (86.4511, 16.388) (86.4452, 17.2152) (86.4406, 18.269) (86.4385, 18.7681) (86.4366, 19.3183) (86.435, 19.92) knots -0.896967 -0.896967 -0.896967 -0.896967 -0.893105 -0.893105 -0.893105 -0.712378 -0.712378 -0.712378 -0.470371 -0.470371 -0.470371 -0.355745 -0.355745 -0.355745 -0.355745
  spline S106 degree 3 poles (39.8457, 55.8029) (39.6452, 55.7934) (39.4421, 55.7811) (39.2359, 55.7654) (38.0093, 55.6721) (36.9931, 55.4584) (36.1486, 55.2305) knots -0.525275 -0.525275 -0.525275 -0.525275 -0.438651 -0.438651 -0.438651 0 0 0 0
  spline S107 degree 3 poles (36.1486, 55.2305) (34.7199, 54.8459) (33.3988, 54.287) (32.2009, 53.6183) (29.9052, 52.3368) (27.7716, 50.5031) (26.1619, 48.0964) knots -0.998654 -0.998654 -0.998654 -0.998654 -0.660747 -0.660747 -0.660747 -0.00186 -0.00186 -0.00186 -0.00186
  spline S108 degree 3 poles (26.1619, 48.0964) (25.7228, 47.443) (25.2558, 46.6787) (24.8304, 45.7931) (24.2651, 44.6161) (23.9062, 43.4937) (23.6465, 42.5142) knots -0.996298 -0.996298 -0.996298 -0.996298 -0.565614 -0.565614 -0.565614 -0.001492 -0.001492 -0.001492 -0.001492
  line L72 (23.6465, 42.5142) -> (23.1572, 40.684)
  line L73 (23.1572, 40.684) -> (23.0983, 15.177)
  spline S109 degree 3 poles (23.0983, 15.177) (23.0312, 14.8729) (22.9604, 14.6077) (22.8935, 14.3903) (22.7847, 14.0364) (22.6726, 13.7909) (22.614, 13.6781) knots -0.942407 -0.942407 -0.942407 -0.942407 -0.737392 -0.737392 -0.737392 -0.374061 -0.374061 -0.374061 -0.374061
  spline S110 degree 3 poles (22.614, 13.6781) (21.2779, 12.1488) (20.2098, 10.3792) (19.5016, 8.433) (18.855, 6.6566) (18.5414, 4.7961) (18.5419, 2.9386) (18.5422, 1.967) (18.6287, 0.9957) (18.8018, 0.0357) (18.9015, -0.5176) (19.03, -1.0671) (19.1876, -1.6105) (19.2621, -1.8673) (19.3431, -2.1227) (19.4306, -2.3764) (19.448, -2.4268) (19.4656, -2.4772) (19.4835, -2.5275) (19.4865, -2.536) (19.4887, -2.5419) (19.4899, -2.5453) (19.4904, -2.5468) (19.4909, -2.5483) (19.4915, -2.5498) knots -0.985418 -0.985418 -0.985418 -0.985418 -0.633646 -0.633646 -0.633646 -0.316442 -0.316442 -0.316442 -0.150537 -0.150537 -0.150537 -0.054917 -0.054917 -0.054917 -0.009736 -0.009736 -0.009736 -0.000758 -0.000758 -0.000758 0.000763 0.000763 0.000763 0.001439 0.001439 0.001439 0.001439
  spline S111 degree 3 poles (19.4915, -2.5498) (19.492, -2.5513) (19.4925, -2.5528) (19.4931, -2.5543) (19.4997, -2.5728) (19.5265, -2.6468) (19.5452, -2.6973) (20.4089, -5.0334) (21.783, -7.047) (23.4444, -8.6564) (25.951, -11.0846) (29.3061, -12.7823) (33.0801, -13.1492) knots -1.001469 -1.001469 -1.001469 -1.001469 -1.000779 -1.000779 -1.000779 -0.992267 -0.992267 -0.992267 -0.598384 -0.598384 -0.598384 -0.000639 -0.000639 -0.000639 -0.000639
  spline S112 degree 3 poles (33.0801, -13.1492) (33.8946, -13.2287) (34.6985, -13.2439) (35.4831, -13.2036) (36.6789, -13.1421) (37.9027, -12.9569) (39.1209, -12.611) (39.8049, -12.4167) (40.4865, -12.1721) (41.1573, -11.8746) (41.5179, -11.7146) (41.8753, -11.5395) (42.2284, -11.3492) (42.3753, -11.27) (42.5215, -11.1882) (42.6668, -11.1038) (42.672, -11.1007) (42.6784, -11.097) (42.6824, -11.0947) knots -1 -1 -1 -1 -0.757667 -0.757667 -0.757667 -0.377854 -0.377854 -0.377854 -0.164598 -0.164598 -0.164598 -0.049947 -0.049947 -0.049947 -0.00224 -0.00224 -0.00224 -0.000531 -0.000531 -0.000531 -0.000531
  spline S113 degree 3 poles (42.6824, -11.0947) (42.7323, -11.0725) (42.9929, -10.971) (43.4558, -10.8919) knots -0.765291 -0.765291 -0.765291 -0.765291 -0.100963 -0.100963 -0.100963 -0.100963
  spline S114 degree 3 poles (43.4558, -10.8919) (43.5537, -10.8888) (43.6864, -10.8852) (43.8603, -10.8817) (44.005, -10.8787) (44.1772, -10.8758) (44.379, -10.8733) (45.1753, -10.8632) (46.4259, -10.8557) (48.3382, -10.8497) (49.4049, -10.8464) (50.6784, -10.8434) (52.1982, -10.8406) (53.2079, -10.8387) (54.3264, -10.8369) (55.5652, -10.8351) (55.8043, -10.8347) (56.0476, -10.8343) (56.2958, -10.834) (56.296, -10.834) (56.2963, -10.834) (56.2965, -10.834) knots -0.740752 -0.740752 -0.740752 -0.740752 -0.65153 -0.65153 -0.65153 -0.57731 -0.57731 -0.57731 -0.288645 -0.288645 -0.288645 -0.127615 -0.127615 -0.127615 -0.020623 -0.020623 -0.020623 0.000021 0.000021 0.000021 0.000039 0.000039 0.000039 0.000039
  spline S115 degree 3 poles (56.2965, -10.834) (56.2967, -10.834) (56.2969, -10.834) (56.2971, -10.834) (57.501, -10.8319) (58.6063, -10.8301) (59.6232, -10.8287) (61.229, -10.8264) (62.6128, -10.8252) (63.807, -10.8253) (66.8776, -10.8257) (68.7239, -10.8388) (69.7618, -10.8605) (70.1491, -10.8685) (70.424, -10.878) (70.5846, -10.886) (70.7089, -10.8921) (70.7851, -10.8968) (70.8187, -10.8992) knots -1.000035 -1.000035 -1.000035 -1.000035 -1.000018 -1.000018 -1.000018 -0.910382 -0.910382 -0.910382 -0.768828 -0.768828 -0.768828 -0.404489 -0.404489 -0.404489 -0.268512 -0.268512 -0.268512 -0.18427 -0.18427 -0.18427 -0.18427
  line L74 (70.8187, -10.8992) -> (70.8682, -10.9067)